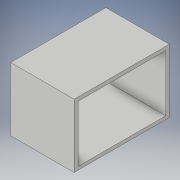
# Autodesk Inventor part: Part3
Saved by Autodesk Inventor 2019 (Build 230136000, 136)
## iProperties
Created: 2019-12-10
Part Number: Part3
Material: Generic
Document SubType Name: Modeling
Designer: ABHISHEK
Density: 1 g/cm^3
Appearance: Default
Author: ABHISHEK
Autodesk Inventor part; units mm, degrees
ref_plane "YZ Plane" through (0, 0, 0) normal (1, 0, 0) x (0, 1, 0)
ref_plane "XZ Plane" through (0, 0, 0) normal (0, 1, 0) x (-1, 0, 0)
ref_plane "XY Plane" through (0, 0, 0) normal (0, 0, 1) x (1, 0, 0)
sketch "Sketch1" plane through (0, 0, 0) normal (1, 0, 0) x (0, 1, 0)
  line L0 (4.4986, 14.2657) -> (-15.5014, 14.2657)
  line L1 (-15.5014, 14.2657) -> (-15.5014, -15.7343)
  line L2 (-15.5014, -15.7343) -> (4.4986, -15.7343)
  line L3 (4.4986, -15.7343) -> (4.4986, 14.2657)
  point P0 (0, 0)
  dimension "d0" = 20
  dimension "d1" = 30
  constraints: 8 end point, 2 parallel, 1 horizontal, 1 perpendicular
  measures "d0" distance of L2.end L1.end
  measures "d1" distance between parallel lines of L2 L0
extrude "Extrusion1" add sketch "Sketch1" along normal blind 20
sketch "Sketch2" plane through (20, 0, 0) normal (1, 0, 0) x (0, 0, -1)
  line L0 (-13.0153, 3.3051) -> (14.6165, 3.3051)
  line L1 (14.6165, 3.3051) -> (14.6165, -14.4728)
  line L2 (14.6165, -14.4728) -> (-13.0153, -14.4728)
  line L3 (-13.0153, -14.4728) -> (-13.0153, 3.3051)
  point P0 (0, 0)
  constraints: 8 end point, 2 parallel, 1 horizontal, 1 perpendicular
extrude "Extrusion2" cut sketch "Sketch2" against normal blind 18
body "Solid1"
